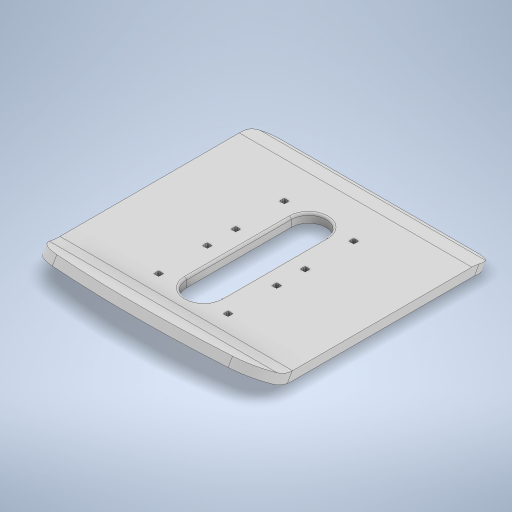
# Autodesk Inventor part: Seat_cutout
Saved by Autodesk Inventor 2023 (Build 270158000, 158)
## iProperties
Created: 2022-10-28
Part Number: Seat_cutout
Material: Generic
Document SubType Name: Modeling
Designer: incep
Density: 1 g/cm^3
Appearance: Default
Author: incep
Autodesk Inventor part; units mm, degrees
ref_plane "YZ Plane" through (0, 0, 0) normal (1, 0, 0) x (0, 1, 0)
ref_plane "XZ Plane" through (0, 0, 0) normal (0, 1, 0) x (-1, 0, 0)
ref_plane "XY Plane" through (0, 0, 0) normal (0, 0, 1) x (1, 0, 0)
sketch "Sketch1" plane through (0, 0, 0) normal (0, 1, 0) x (-1, 0, 0)
  line L0 (55, -48) -> (-55, -48) construction
  line L1 (-60, -43) -> (-60, 43) construction
  line L2 (-55, 48) -> (55, 48) construction
  line L3 (60, 43) -> (60, -43) construction
  line L4 (50, -35) -> (-50, -35) construction
  line L5 (-50, -35) -> (-50, 35) construction
  line L6 (-50, 35) -> (50, 35) construction
  line L7 (50, 35) -> (50, -35) construction
  arc A0 (60, 43) -> (55, 48) centre (55, 43) ccw construction
  arc A1 (-55, 48) -> (-60, 43) centre (-55, 43) ccw construction
  arc A2 (-60, -43) -> (-55, -48) centre (-55, -43) ccw construction
  arc A3 (55, -48) -> (60, -43) centre (55, -43) ccw construction
  circle A4 centre (-50, 35) radius 3.4 construction
  line L8 (0, -20) -> (0, 20) construction
  line L9 (25, -20) -> (25, 20) construction
  line L10 (-25, 20) -> (-25, -20) construction
  arc A5 (-25, -20) -> (25, -20) centre (0, -20) ccw construction
  arc A6 (25, 20) -> (-25, 20) centre (0, 20) ccw construction
  line L11 (55, -159) -> (-55, -159) construction
  line L12 (-60, -154) -> (-60, -68) construction
  line L13 (-55, -63) -> (55, -63) construction
  line L14 (60, -68) -> (60, -154) construction
  line L15 (50, -146) -> (-50, -146) construction
  line L16 (-50, -146) -> (-50, -76) construction
  line L17 (-50, -76) -> (50, -76) construction
  line L18 (50, -76) -> (50, -146) construction
  arc A7 (60, -68) -> (55, -63) centre (55, -68) ccw construction
  arc A8 (-55, -63) -> (-60, -68) centre (-55, -68) ccw construction
  arc A9 (-60, -154) -> (-55, -159) centre (-55, -154) ccw construction
  arc A10 (55, -159) -> (60, -154) centre (55, -154) ccw construction
  line L19 (0, -131) -> (0, -91) construction
  line L20 (25, -131) -> (25, -91) construction
  line L21 (-25, -91) -> (-25, -131) construction
  arc A11 (-25, -131) -> (25, -131) centre (0, -131) ccw construction
  arc A12 (25, -91) -> (-25, -91) centre (0, -91) ccw construction
  line L22 (0, -131) -> (0, 20) construction
  line L23 (25, -131) -> (25, 20)
  line L24 (-25, 20) -> (-25, -131)
  arc A13 (-25, -131) -> (25, -131) centre (0, -131) ccw
  arc A14 (25, 20) -> (-25, 20) centre (0, 20) ccw
  line L25 (167.5, -187) -> (-167.5, -187)
  line L26 (-167.5, -187) -> (-167.5, 48)
  line L27 (-167.5, 48) -> (167.5, 48)
  line L28 (167.5, 48) -> (167.5, -187)
  line L29 (-53.5, 38.5) -> (-51.3463, 38.5)
  line L30 (-48.6537, 38.5) -> (-46.5, 38.5)
  arc A15 (-48.6537, 38.5) -> (-51.3463, 38.5) centre (-50, 35) ccw
  line L31 (-46.5, 38.5) -> (-46.5, 36.3463)
  line L32 (-46.5, 33.6537) -> (-46.5, 31.5)
  arc A16 (-46.5, 33.6537) -> (-46.5, 36.3463) centre (-50, 35) ccw
  line L33 (-46.5, 31.5) -> (-48.6537, 31.5)
  line L34 (-51.3463, 31.5) -> (-53.5, 31.5)
  arc A17 (-53.5, 36.3463) -> (-53.5, 33.6537) centre (-50, 35) ccw
  arc A18 (-51.3463, 31.5) -> (-48.6537, 31.5) centre (-50, 35) ccw
  line L35 (-53.5, 31.5) -> (-53.5, 33.6537)
  line L36 (-53.5, 36.3463) -> (-53.5, 38.5)
  circle A19 centre (-50, 35) radius 3.75 construction
  line L37 (-53.5, 38.5) -> (-53.5, 31.5) construction
  line L38 (-53.5, 38.5) -> (-46.5, 38.5) construction
  line L39 (-46.5, 31.5) -> (-53.5, 31.5) construction
  line L40 (-46.5, 38.5) -> (-46.5, 31.5) construction
  circle A20 centre (50, 35) radius 3.4 construction
  arc A21 (51.3463, 38.5) -> (48.6537, 38.5) centre (50, 35) ccw
  line L41 (46.5, 36.3463) -> (46.5, 38.5)
  line L42 (53.5, 38.5) -> (53.5, 36.3463)
  arc A22 (53.5, 33.6537) -> (53.5, 36.3463) centre (50, 35) ccw
  line L43 (46.5, 38.5) -> (46.5, 31.5) construction
  line L44 (53.5, 38.5) -> (53.5, 31.5) construction
  circle A23 centre (50, 35) radius 3.75 construction
  line L45 (53.5, 33.6537) -> (53.5, 31.5)
  line L46 (53.5, 31.5) -> (51.3463, 31.5)
  line L47 (53.5, 31.5) -> (46.5, 31.5) construction
  arc A24 (48.6537, 31.5) -> (51.3463, 31.5) centre (50, 35) ccw
  line L48 (48.6537, 31.5) -> (46.5, 31.5)
  line L49 (46.5, 31.5) -> (46.5, 33.6537)
  arc A25 (46.5, 36.3463) -> (46.5, 33.6537) centre (50, 35) ccw
  line L50 (46.5, 38.5) -> (48.6537, 38.5)
  line L51 (51.3463, 38.5) -> (53.5, 38.5)
  line L52 (46.5, 38.5) -> (53.5, 38.5) construction
  circle A26 centre (-50, -35) radius 3.4 construction
  arc A27 (-48.6537, -31.5) -> (-51.3463, -31.5) centre (-50, -35) ccw
  line L53 (-53.5, -33.6537) -> (-53.5, -31.5)
  line L54 (-46.5, -31.5) -> (-46.5, -33.6537)
  arc A28 (-46.5, -36.3463) -> (-46.5, -33.6537) centre (-50, -35) ccw
  line L55 (-53.5, -31.5) -> (-53.5, -38.5) construction
  line L56 (-46.5, -31.5) -> (-46.5, -38.5) construction
  circle A29 centre (-50, -35) radius 3.75 construction
  line L57 (-46.5, -36.3463) -> (-46.5, -38.5)
  line L58 (-46.5, -38.5) -> (-48.6537, -38.5)
  line L59 (-46.5, -38.5) -> (-53.5, -38.5) construction
  arc A30 (-51.3463, -38.5) -> (-48.6537, -38.5) centre (-50, -35) ccw
  line L60 (-51.3463, -38.5) -> (-53.5, -38.5)
  line L61 (-53.5, -38.5) -> (-53.5, -36.3463)
  arc A31 (-53.5, -33.6537) -> (-53.5, -36.3463) centre (-50, -35) ccw
  line L62 (-53.5, -31.5) -> (-51.3463, -31.5)
  line L63 (-48.6537, -31.5) -> (-46.5, -31.5)
  line L64 (-53.5, -31.5) -> (-46.5, -31.5) construction
  circle A32 centre (50, -35) radius 3.4 construction
  arc A33 (51.3463, -31.5) -> (48.6537, -31.5) centre (50, -35) ccw
  line L65 (46.5, -33.6537) -> (46.5, -31.5)
  line L66 (53.5, -31.5) -> (53.5, -33.6537)
  arc A34 (53.5, -36.3463) -> (53.5, -33.6537) centre (50, -35) ccw
  line L67 (46.5, -31.5) -> (46.5, -38.5) construction
  line L68 (53.5, -31.5) -> (53.5, -38.5) construction
  circle A35 centre (50, -35) radius 3.75 construction
  line L69 (53.5, -36.3463) -> (53.5, -38.5)
  line L70 (53.5, -38.5) -> (51.3463, -38.5)
  line L71 (53.5, -38.5) -> (46.5, -38.5) construction
  arc A36 (48.6537, -38.5) -> (51.3463, -38.5) centre (50, -35) ccw
  line L72 (48.6537, -38.5) -> (46.5, -38.5)
  line L73 (46.5, -38.5) -> (46.5, -36.3463)
  arc A37 (46.5, -33.6537) -> (46.5, -36.3463) centre (50, -35) ccw
  line L74 (46.5, -31.5) -> (48.6537, -31.5)
  line L75 (51.3463, -31.5) -> (53.5, -31.5)
  line L76 (46.5, -31.5) -> (53.5, -31.5) construction
  circle A38 centre (-50, -76) radius 3.4 construction
  line L77 (-53.5, -72.5) -> (-51.3463, -72.5)
  line L78 (-48.6537, -72.5) -> (-46.5, -72.5)
  arc A39 (-48.6537, -72.5) -> (-51.3463, -72.5) centre (-50, -76) ccw
  line L79 (-46.5, -72.5) -> (-46.5, -74.6537)
  line L80 (-46.5, -77.3463) -> (-46.5, -79.5)
  arc A40 (-46.5, -77.3463) -> (-46.5, -74.6537) centre (-50, -76) ccw
  line L81 (-46.5, -79.5) -> (-48.6537, -79.5)
  line L82 (-51.3463, -79.5) -> (-53.5, -79.5)
  arc A41 (-53.5, -74.6537) -> (-53.5, -77.3463) centre (-50, -76) ccw
  arc A42 (-51.3463, -79.5) -> (-48.6537, -79.5) centre (-50, -76) ccw
  line L83 (-53.5, -79.5) -> (-53.5, -77.3463)
  line L84 (-53.5, -74.6537) -> (-53.5, -72.5)
  circle A43 centre (-50, -76) radius 3.75 construction
  line L85 (-53.5, -72.5) -> (-53.5, -79.5) construction
  line L86 (-53.5, -72.5) -> (-46.5, -72.5) construction
  line L87 (-46.5, -79.5) -> (-53.5, -79.5) construction
  line L88 (-46.5, -72.5) -> (-46.5, -79.5) construction
  arc A44 (53.5, -77.3463) -> (53.5, -74.6537) centre (50, -76) ccw
  line L89 (53.5, -77.3463) -> (53.5, -79.5)
  line L90 (53.5, -79.5) -> (51.3463, -79.5)
  line L91 (53.5, -72.5) -> (53.5, -74.6537)
  line L92 (53.5, -72.5) -> (53.5, -79.5) construction
  line L93 (51.3463, -72.5) -> (53.5, -72.5)
  line L94 (53.5, -79.5) -> (46.5, -79.5) construction
  arc A45 (51.3463, -72.5) -> (48.6537, -72.5) centre (50, -76) ccw
  circle A46 centre (50, -76) radius 3.4 construction
  line L95 (46.5, -72.5) -> (53.5, -72.5) construction
  circle A47 centre (50, -76) radius 3.75 construction
  line L96 (46.5, -72.5) -> (46.5, -79.5) construction
  line L97 (46.5, -72.5) -> (48.6537, -72.5)
  line L98 (46.5, -74.6537) -> (46.5, -72.5)
  arc A48 (46.5, -74.6537) -> (46.5, -77.3463) centre (50, -76) ccw
  line L99 (46.5, -79.5) -> (46.5, -77.3463)
  line L100 (48.6537, -79.5) -> (46.5, -79.5)
  arc A49 (48.6537, -79.5) -> (51.3463, -79.5) centre (50, -76) ccw
  arc A50 (-46.5, -147.3463) -> (-46.5, -144.6537) centre (-50, -146) ccw
  line L101 (-46.5, -147.3463) -> (-46.5, -149.5)
  line L102 (-46.5, -149.5) -> (-48.6537, -149.5)
  line L103 (-46.5, -142.5) -> (-46.5, -144.6537)
  line L104 (-46.5, -142.5) -> (-46.5, -149.5) construction
  line L105 (-48.6537, -142.5) -> (-46.5, -142.5)
  line L106 (-46.5, -149.5) -> (-53.5, -149.5) construction
  arc A51 (-48.6537, -142.5) -> (-51.3463, -142.5) centre (-50, -146) ccw
  circle A52 centre (-50, -146) radius 3.4 construction
  line L107 (-53.5, -142.5) -> (-46.5, -142.5) construction
  circle A53 centre (-50, -146) radius 3.75 construction
  line L108 (-53.5, -142.5) -> (-53.5, -149.5) construction
  line L109 (-53.5, -142.5) -> (-51.3463, -142.5)
  line L110 (-53.5, -144.6537) -> (-53.5, -142.5)
  arc A54 (-53.5, -144.6537) -> (-53.5, -147.3463) centre (-50, -146) ccw
  line L111 (-53.5, -149.5) -> (-53.5, -147.3463)
  line L112 (-51.3463, -149.5) -> (-53.5, -149.5)
  arc A55 (-51.3463, -149.5) -> (-48.6537, -149.5) centre (-50, -146) ccw
  arc A56 (53.5, -147.3463) -> (53.5, -144.6537) centre (50, -146) ccw
  line L113 (53.5, -147.3463) -> (53.5, -149.5)
  line L114 (53.5, -149.5) -> (51.3463, -149.5)
  line L115 (53.5, -142.5) -> (53.5, -144.6537)
  line L116 (53.5, -142.5) -> (53.5, -149.5) construction
  line L117 (51.3463, -142.5) -> (53.5, -142.5)
  line L118 (53.5, -149.5) -> (46.5, -149.5) construction
  arc A57 (51.3463, -142.5) -> (48.6537, -142.5) centre (50, -146) ccw
  circle A58 centre (50, -146) radius 3.4 construction
  line L119 (46.5, -142.5) -> (53.5, -142.5) construction
  circle A59 centre (50, -146) radius 3.75 construction
  line L120 (46.5, -142.5) -> (46.5, -149.5) construction
  line L121 (46.5, -142.5) -> (48.6537, -142.5)
  line L122 (46.5, -144.6537) -> (46.5, -142.5)
  arc A60 (46.5, -144.6537) -> (46.5, -147.3463) centre (50, -146) ccw
  line L123 (46.5, -149.5) -> (46.5, -147.3463)
  line L124 (48.6537, -149.5) -> (46.5, -149.5)
  arc A61 (48.6537, -149.5) -> (51.3463, -149.5) centre (50, -146) ccw
  point P0 (0, 0)
  point P1 (-60, 0)
  point P2 (0, -48)
  point P3 (0, -35)
  point P4 (-50, 0)
  point P5 (0, 0)
  point P6 (0, -111)
  point P7 (-60, -111)
  point P8 (0, -159)
  point P9 (0, -146)
  point P10 (-50, -111)
  point P11 (0, -111)
  point P12 (0, -55.5)
  point P13 (0, 48)
  point P14 (-53.5, 35)
  point P15 (-50, 38.5)
  point P16 (46.5, 35)
  point P17 (50, 38.5)
  point P18 (-53.5, -35)
  point P19 (-50, -31.5)
  point P20 (46.5, -35)
  point P21 (50, -31.5)
  point P22 (-53.5, -76)
  point P23 (-50, -72.5)
  point P24 (50, -72.5)
  point P25 (46.5, -76)
  point P26 (-50, -142.5)
  point P27 (-53.5, -146)
  point P28 (50, -142.5)
  point P29 (46.5, -146)
  dimension "d0" = 96
  dimension "d1" = 120
  dimension "d2" = 70
  dimension "d3" = 100
  dimension "d4" = 5
  dimension "d10" = 6.8
  dimension "d13" = 25
  dimension "d14" = 40
  dimension "d17" = 96
  dimension "d18" = 120
  dimension "d19" = 70
  dimension "d20" = 100
  dimension "d21" = 5
  dimension "d26" = 25
  dimension "d27" = 40
  dimension "d36" = 15
  dimension "d37" = 235
  dimension "d38" = 335
  dimension "d39" = 0
  dimension "d64" = 7
  dimension "d65" = 7
  dimension "d66" = 7.5
  dimension "d69" = 100
  dimension "d72" = 70
  dimension "d75" = 6.8
  dimension "d76" = 7
  dimension "d77" = 7
  dimension "d78" = 7.5
  dimension "d84" = 100
  dimension "d87" = 70
  constraints: 256 end point, 92 point on circle, 62 centre point, 36 tangent, 30 coincident, 29 parallel, 16 midpoint, 16 perpendicular, 12 collinear, 11 horizontal, 8 vertical alignment, 6 equal radius, 6 horizontal alignment, 6 vertical, 219 other
  measures "d0" distance between parallel lines of L2 L0
  measures "d1" distance between parallel lines of L1 L3
  measures "d2" distance between parallel lines of L6 L4
  measures "d3" distance between parallel lines of L7 L5
  measures "d4" radius of A0
  measures "d10" diameter of A4
  measures "d13" radius of A5
  measures "d14" distance of L8.end L8.start
  measures "d17" distance between parallel lines of L13 L11
  measures "d18" distance between parallel lines of L12 L14
  measures "d19" distance between parallel lines of L17 L15
  measures "d20" distance between parallel lines of L18 L16
  measures "d21" radius of A7
  measures "d26" radius of A11
  measures "d27" distance of L19.end L19.start
  measures "d36" distance between parallel lines of L0 L13
  measures "d37" distance of L25.end L26.end
  measures "d38" distance of L26.end L27.end
  measures "d39" distance between parallel lines of L27 L2
  measures "d64" distance of L34.end L29.start
  measures "d65" distance of L30.end L29.start
  measures "d66" diameter of A19
  measures "d69" distance of L5.end point (50, 35)
  measures "d72" distance of L5.end point (-50, -35)
  measures "d75" diameter of A38
  measures "d76" distance of L82.end L77.start
  measures "d77" distance of L78.end L77.start
  measures "d78" diameter of A43
  measures "d84" distance of L16.end point (50, -76)
  measures "d87" distance of L16.end point (-50, -146)
extrude "Extrusion1" add sketch "Sketch1" along normal blind 12.7
sketch "Sketch2" plane through (167.5, 0, 48) normal (1, 0, 0) x (0, 0, -1)
  line L0 (0, 0) -> (0, 12.7) construction
  line L1 (0, 0) -> (-25, 0) construction
  line L2 (-25, 0) -> (-75, 28.8675) construction
  line L3 (0, 12.7) -> (-21.597, 12.7) construction
  line L4 (-21.597, 12.7) -> (-68.65, 39.866) construction
  line L5 (-75, 28.8675) -> (-68.65, 39.866) construction
  line L6 (0, 12.7) -> (0, 0)
  line L7 (0, 0) -> (-11.6025, 0)
  line L8 (-36.6025, 6.6987) -> (-75, 28.8675)
  line L9 (-75, 28.8675) -> (-68.65, 39.866)
  line L10 (-68.65, 39.866) -> (-30.2525, 17.6973)
  line L11 (-11.6025, 12.7) -> (0, 12.7)
  arc A0 (-36.6025, 6.6987) -> (-11.6025, 0) centre (-11.6025, 50) ccw
  arc A1 (-30.2525, 17.6973) -> (-11.6025, 12.7) centre (-11.6025, 50) ccw
  point P0 (48, 0)
  dimension "d40" = 30
  dimension "d41" = 12.7
  dimension "d42" = 75
  dimension "d43" = 25
  dimension "d44" = 50
  dimension "d45" = 37.3
  constraints: 22 end point, 4 collinear, 4 point on circle, 4 point on line, 4 tangent, 2 centre point, 2 horizontal, 2 perpendicular, 1 parallel, 1 vertical
  measures "d40" angle of L2 L1
  measures "d41" distance of L2.end L4.end
  measures "d42" horizontal distance of L2.end L0.start
  measures "d43" distance of L0.start L1.end
  measures "d44" radius of A0
  measures "d45" radius of A1
extrude "Extrusion2" add sketch "Sketch2" against normal up to surface (335 mm away)
fillet "Fillet1" [suppressed]
fillet "Fillet2" [suppressed]
sketch "Sketch3" plane through (167.5, 0, -187) normal (1, 0, 0) x (0, 0, -1)
  line L0 (0, 0) -> (-246.6025, 0) construction
  line L1 (0, 0) -> (21.597, 0) construction
  line L2 (21.597, 0) -> (38.65, -9.8455) construction
  line L3 (38.65, -9.8455) -> (45, 1.153) construction
  line L4 (45, 1.153) -> (25, 12.7) construction
  line L5 (0, 0) -> (0, 12.7) construction
  line L6 (25, 12.7) -> (0, 12.7) construction
  line L7 (-246.6025, 0) -> (0, 0) projected
  line L8 (0, 0) -> (0, 12.7)
  line L9 (0, 12.7) -> (-246.6025, 12.7) projected
  line L10 (0, 12.7) -> (11.6025, 12.7)
  line L11 (36.6025, 6.0013) -> (45, 1.153)
  line L12 (45, 1.153) -> (38.65, -9.8455)
  line L13 (38.65, -9.8455) -> (30.2525, -4.9973)
  line L14 (11.6025, 0) -> (0, 0)
  arc A0 (36.6025, 6.0013) -> (11.6025, 12.7) centre (11.6025, -37.3) ccw
  arc A1 (30.2525, -4.9973) -> (11.6025, 0) centre (11.6025, -37.3) ccw
  point P0 (-187, 0)
  point P1 (-260.5983, 0)
  point P2 (-256.5569, 7)
  point P3 (-235, 0)
  dimension "d50" = 12.7
  dimension "d51" = 25
  dimension "d52" = 30
  dimension "d53" = 45
  dimension "d54" = 50
  dimension "d55" = 37.3
  constraints: 22 end point, 4 perpendicular, 4 point on circle, 4 point on line, 4 tangent, 3 parallel, 2 centre point, 2 horizontal, 1 collinear, 1 other
  measures "d50" distance of L2.end L3.end
  measures "d51" distance of L4.end L5.end
  measures "d52" angle of L4 L6
  measures "d53" horizontal distance of L3.end L5.end
  measures "d54" radius of A0
  measures "d55" radius of A1
extrude "Extrusion3" add sketch "Sketch3" against normal up to surface (335 mm away)
fillet "Fillet3" radius 25 2 edges at (167.5, -4.3463, -228.825) (-167.5, -4.3463, -228.825)
sketch "Sketch4" plane through (-167.5, 39.866, 116.65) normal (0, 0.8660254, -0.5) x (1, 0, 0)
  line L0 (335, 44.3376) -> (335, 0) construction
  line L1 (335, 22.1688) -> (0, 22.1688) construction
  line L2 (0, 44.3376) -> (0, 0) construction
  arc A0 (0, 22.1688) -> (335, 22.1688) centre (167.5, 696.8782) ccw
  line L3 (335, 22.1688) -> (335, 0)
  line L4 (335, 0) -> (0, 0) projected
  line L5 (335, 0) -> (0, 0)
  line L6 (0, 0) -> (0, 22.1688)
  point P0 (167.5, 120.9549)
  constraints: 8 end point, 2 horizontal, 2 midpoint, 2 point on circle, 1 centre point, 1 perpendicular, 1 vertical
extrude "Extrusion4" cut sketch "Sketch4" against normal up to surface (12.7 mm away)
fillet "Fillet4" radius 50 2 edges at (167.5, 23.2824, 100.6263) (-167.5, 23.2824, 100.6263)
fillet "Fillet5" radius 3 4 edges at (0, 12.7, -156) (25, 12.7, -55.5) (0, 12.7, 45) (-25, 12.7, -55.5)
sketch "LaserCuttingGuide" plane through (0, 0, 0) normal (0, -1, 0) x (1, 0, 0)
  line L0 (-60, 43) -> (-60, -43) construction
  line L1 (-55, -48) -> (55, -48) construction
  line L2 (60, -43) -> (60, 43) construction
  line L3 (55, 48) -> (-55, 48) construction
  line L4 (55, -63) -> (-55, -63) construction
  line L5 (-60, -68) -> (-60, -154) construction
  line L6 (60, -154) -> (60, -68) construction
  line L7 (-55, -159) -> (55, -159) construction
  line L8 (-60, 48) -> (60, 48)
  line L9 (60, 48) -> (60, -48)
  line L10 (-60, -48) -> (-60, 48)
  line L11 (60, -63) -> (60, -159)
  line L12 (60, -159) -> (-60, -159)
  line L13 (-60, -159) -> (-60, -63)
  line L14 (5.3292, -48) -> (5.3292, -63)
  line L15 (-7.209, -63) -> (-7.209, -48)
  line L16 (-60, -63) -> (-7.209, -63)
  line L17 (5.3292, -63) -> (60, -63)
  line L18 (60, -48) -> (5.3292, -48)
  line L19 (-7.209, -48) -> (-60, -48)
  point P0 (0, 0)
  constraints: 24 end point, 10 collinear, 7 parallel, 3 horizontal, 3 perpendicular
extrude "Extrusion5" [suppressed]
equation "\"d0\" = moduleHeight"
equation "\"d1\" = moduleWidth"
equation "\"d2\" = moduleMountH"
equation "\"d3\" = moduleMountW"
equation "\"d4\" = moduleCornerR"
equation "\"d10\" = moduleMountD"
equation "\"d13\" = moduleOpeningR"
equation "\"d14\" = moduleOpeningH"
equation "\"d17\" = d28"
equation "\"d18\" = d29"
equation "\"d19\" = d30"
equation "\"d20\" = d31"
equation "\"d21\" = d32"
equation "\"d26\" = d34"
equation "\"d27\" = d35"
equation "\"d36\" = moduleSpacing"
equation "\"d37\" = seatFlatH"
equation "\"d38\" = seatW"
equation "\"d64\" = carriageM6neck"
equation "\"d15\" = thickness"
equation "\"d40\" = seatA"
equation "\"d41\" = thickness"
equation "\"d42\" = seatBackExtension"
equation "\"d43\" = 0.5 * seatExtensionOuterR"
equation "\"d44\" = seatExtensionOuterR"
equation "\"d45\" = seatExtensionOuterR - thickness"
equation "\"d46\" = thickness"
equation "\"d50\" = thickness"
equation "\"d51\" = 0.5 * seatExtensionOuterR"
equation "\"d52\" = seatA"
equation "\"d53\" = seatFrontExtension"
equation "\"d54\" = seatExtensionOuterR"
equation "\"d55\" = seatExtensionOuterR - thickness"
equation "\"moduleWidth\" = 120"
equation "\"moduleHeight\" = 96"
equation "\"moduleMountW\" = 100"
equation "\"moduleMountH\" = 70"
equation "\"moduleMountD\" = 6.8"
equation "\"moduleCornerR\" = 5"
equation "\"moduleOpeningR\" = 25"
equation "\"moduleOpeningH\" = 40"
equation "\"thickness\" = 12.7"
equation "\"d28\" = 96"
equation "\"d29\" = 120"
equation "\"d30\" = 70"
equation "\"d31\" = 100"
equation "\"d32\" = 5"
equation "\"d33\" = 6.8"
equation "\"d34\" = 25"
equation "\"d35\" = 40"
equation "\"moduleSpacing\" = 15"
equation "\"seatFlatH\" = 235"
equation "\"seatW\" = 335"
equation "\"moduleRearMargin\" = 0"
equation "\"seatA\" = 30deg"
equation "\"seatBackExtension\" = 75"
equation "\"seatExtensionOuterR\" = 50"
equation "\"seatFrontExtension\" = 45"
equation "\"carriageM6neck\" = 7"
equation "\"insertM6D\" = 7.5"
equation "\"d63\" = insertM6D"
equation "\"d79\" = 6.8"
equation "\"d80\" = 7"
equation "\"d81\" = 7.5"
body "Solid1"
